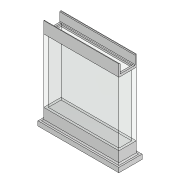
# Autodesk Inventor part: Box
Saved by Autodesk Inventor 2021 (Build 250183000, 183)
## iProperties
Created: 2021-04-01
Part Number: Box
Material: Generic
Document SubType Name: Modeling
Designer: Tran Duc Viet
Mass: 4223.94 g
Surface Area: 6399.34 cm^2
Volume: 4223.94 cm^3
Density: 1 g/cm^3
Appearance: Default
Author: Tran Duc Viet
Autodesk Inventor part; units mm, degrees
ref_plane "YZ Plane" through (0, 0, 0) normal (1, 0, 0) x (0, 1, 0)
sketch "Sketch1" plane through (0, 0, 0) normal (0, 1, 0) x (-1, 0, 0)
  line L0 (152.5, 27.5) -> (-152.5, 27.5)
  line L1 (-152.5, 27.5) -> (-152.5, -27.5)
  line L2 (-152.5, -27.5) -> (152.5, -27.5)
  line L3 (152.5, -27.5) -> (152.5, 27.5)
  line L4 (152.5, 27.5) -> (-152.5, -27.5) construction
  line L5 (-152.5, 27.5) -> (152.5, -27.5) construction
  line L6 (162.5, 37.5) -> (-162.5, 37.5)
  line L7 (-162.5, 37.5) -> (-162.5, -37.5)
  line L8 (-162.5, -37.5) -> (162.5, -37.5)
  line L9 (162.5, -37.5) -> (162.5, 37.5)
  line L10 (162.5, 37.5) -> (-162.5, -37.5) construction
  line L11 (-162.5, 37.5) -> (162.5, -37.5) construction
  point P0 (0, 0)
  dimension "d0" = 305
  dimension "d1" = 55
  dimension "d2" = 325
  dimension "d3" = 75
  constraints: 24 end point, 4 midpoint, 4 parallel, 2 horizontal, 2 perpendicular
  measures "d0" distance of L2.end L1.end
  measures "d1" distance of L1.end L0.end
  measures "d2" distance of L8.end L7.end
  measures "d3" distance of L8.end L6.start
extrude "Extrusion1" add sketch "Sketch1" along normal blind 325
ref_plane "Work Plane1" through (0, 275, 0) normal (0, 1, 0) x (1, 0, 0)
sketch "Sketch2" plane through (0, 0, 0) normal (0, -1, 0) x (1, 0, 0)
  line L0 (162.5, 37.5) -> (162.5, -37.5) projected
  line L1 (-162.5, -37.5) -> (162.5, -37.5)
  line L2 (162.5, -37.5) -> (162.5, 37.5)
  line L3 (162.5, 37.5) -> (-162.5, 37.5)
  line L4 (-162.5, 37.5) -> (-162.5, -37.5)
  line L5 (-162.5, -37.5) -> (162.5, 37.5) construction
  line L6 (162.5, -37.5) -> (-162.5, 37.5) construction
  point P0 (0, 0)
  constraints: 12 end point, 2 midpoint, 2 parallel, 1 horizontal, 1 perpendicular
extrude "Extrusion2" add sketch "Sketch2" along normal blind 50
sketch "Sketch3" plane through (0, -50, 0) normal (0, -1, 0) x (1, 0, 0)
  line L0 (-175, -50) -> (175, -50)
  line L1 (175, -50) -> (175, 50)
  line L2 (175, 50) -> (-175, 50)
  line L3 (-175, 50) -> (-175, -50)
  line L4 (-175, -50) -> (175, 50) construction
  line L5 (175, -50) -> (-175, 50) construction
  point P0 (0, 0)
  dimension "d9" = 350
  dimension "d10" = 100
  constraints: 12 end point, 2 midpoint, 2 parallel, 1 horizontal, 1 perpendicular
  measures "d9" distance of L2.end L1.end
  measures "d10" distance of L1.end L0.end
extrude "Extrusion3" add sketch "Sketch3" along normal blind 20
chamfer "Chamfer2" distance 5 angle 45 4 edges at (0, 325, -27.5) (-152.5, 325, 0) (0, 325, 27.5) (152.5, 325, 0)
split body "Split1" result two bodies by plane through (0, 275, 0) normal (0, 1, 0) first body at (54.1667, 308.3333, -37)
ref_plane "Work Plane2" through (0, 0, 0) normal (0, -1, 0) x (1, 0, 0)
split body "Split2" result two bodies by plane through (0, 0, 0) normal (0, -1, 0) bodies 3 first body at (58.3333, -69.5, -16.6667)
chamfer "Chamfer4" distance 5 angle 45 4 edges at (0, -50, 37.5) (162.5, -50, 0) (-162.5, -50, 0) (0, -50, -37.5)
sketch "Sketch10" plane through (0, 325, 0) normal (0, 1, 0) x (1, 0, 0)
  line L0 (-167.5, 42.5) -> (-167.5, -42.5) projected
  line L1 (167.5, -42.5) -> (167.5, 42.5) projected
  line L2 (-167.5, 32.5) -> (167.5, 32.5)
  line L3 (167.5, 32.5) -> (167.5, -32.5)
  line L4 (167.5, -32.5) -> (-167.5, -32.5)
  line L5 (-167.5, -32.5) -> (-167.5, 32.5)
  line L6 (-167.5, -42.5) -> (167.5, -42.5) projected
  line L7 (167.5, 42.5) -> (-167.5, 42.5) projected
  point P0 (0, 0)
  point P1 (-167.5, -32.5)
  dimension "d53" = 10
  dimension "d54" = 10
  constraints: 8 end point, 2 parallel, 2 point on line, 1 horizontal, 1 perpendicular
  measures "d53" distance between parallel lines of L6 L4
  measures "d54" distance between parallel lines of L7 L2
extrude "Extrusion7" cut sketch "Sketch10" against normal blind 40 contours L2 L1 L4 L0 bodies 2
fillet "Fillet1" radius 2.5 8 edges at (0, 285, -27.5) (-152.5, 285, 0) (0, 285, 27.5) (152.5, 285, 0) (0, 285, -32.5) (0, 285, 32.5) (0, 325, 32.5) (0, 325, -32.5)
equation "\"d4\" = d2"
